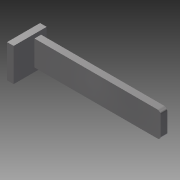
# Autodesk Inventor part: Powerpole45APCBStraight
Saved by Autodesk Inventor 2014 SP1 (Build 180222100, 222)
## iProperties
Created: 2016-03-18
Part Number: Powerpole45APCBStraight
Material: Stainless Steel
Document SubType Name: Modeling
Designer: Tyler
Density: 8.08 g/cm^3
Appearance: Semi-Polished
Author: Tyler
Autodesk Inventor part; units mm, degrees
ref_plane "YZ Plane" through (0, 0, 0) normal (1, 0, 0) x (0, 1, 0)
ref_plane "XZ Plane" through (0, 0, 0) normal (0, 1, 0) x (-1, 0, 0)
ref_plane "XY Plane" through (0, 0, 0) normal (0, 0, 1) x (1, 0, 0)
sketch "Sketch1" plane through (0, 0, 0) normal (0, 1, 0) x (-1, 0, 0)
  line L0 (-10.05, -1.9) -> (10.05, -1.9)
  line L1 (10.05, -1.9) -> (10.05, 1.9)
  line L2 (10.05, 1.9) -> (-10.05, 1.9)
  line L3 (-10.05, 1.9) -> (-10.05, -1.9)
  line L4 (-10.05, -1.9) -> (10.05, 1.9) construction
  line L5 (10.05, -1.9) -> (-10.05, 1.9) construction
  point P0 (0, 0)
  dimension "d0" = 3.8
  dimension "d1" = 20.1
  constraints: 12 end point, 2 midpoint, 2 parallel, 1 horizontal, 1 perpendicular
  measures "d0" distance of L2.end L0.start
  measures "d1" distance of L1.end L2.end
extrude "Extrusion1" add sketch "Sketch1" along normal blind 1
fillet "Fillet1" radius 0.5 2 edges at (10.05, 0.5, 1.9) (10.05, 0.5, -1.9)
sketch "Sketch2" plane through (-10.05, 0, -1.9) normal (-1, 0, 0) x (0, 0, 1)
  line L0 (0, 0) -> (3.8, 0) projected
  line L1 (3.8, 0) -> (3.8, 1) projected
  line L2 (0, 1) -> (3.8, 1) projected
  line L3 (0, 0) -> (0, 1) projected
  line L4 (-0.6, -3.15) -> (4.4, -3.15)
  line L5 (4.4, -3.15) -> (4.4, 1.85)
  line L6 (4.4, 1.85) -> (-0.6, 1.85)
  line L7 (-0.6, 1.85) -> (-0.6, -3.15)
  line L8 (-0.6, -3.15) -> (4.4, 1.85) construction
  line L9 (4.4, -3.15) -> (-0.6, 1.85) construction
  line L10 (-2.05, -4.6) -> (5.85, -4.6) construction
  line L11 (5.85, -4.6) -> (5.85, 3.3) construction
  line L12 (5.85, 3.3) -> (-2.05, 3.3) construction
  line L13 (-2.05, 3.3) -> (-2.05, -4.6) construction
  line L14 (-2.05, -4.6) -> (5.85, 3.3) construction
  line L15 (5.85, -4.6) -> (-2.05, 3.3) construction
  point P0 (1.9, 0)
  point P1 (1.9, -0.65)
  point P2 (1.9, -0.65)
  dimension "d5" = 5
  dimension "d6" = 5
  dimension "d7" = 7.9
  dimension "d8" = 7.9
  dimension "d9" = 3.3
  dimension "d10" = 2.5
  constraints: 24 end point, 5 midpoint, 4 parallel, 2 horizontal, 2 perpendicular
  measures "d5" distance of L6.end L5.end
  measures "d6" distance of L5.end L4.end
  measures "d7" distance of L12.end L11.end
  measures "d8" distance of L11.end L10.end
  measures "d9" distance between parallel lines of L0 L12
  measures "d10" distance from line of L7 point (1.9, 0)
extrude "Extrusion2" add sketch "Sketch2" against normal blind 1
body "Solid1"
